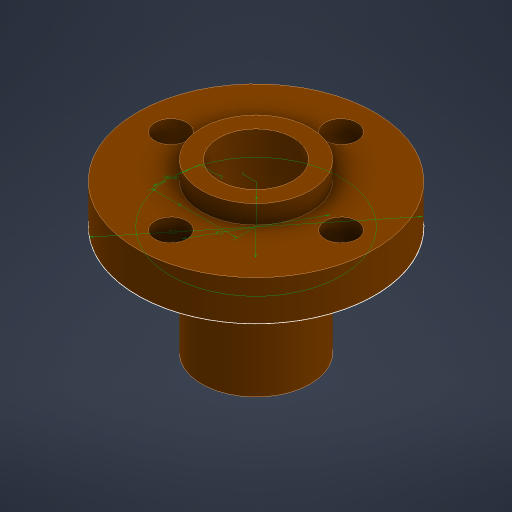
# Autodesk Inventor part: Leadscrew
Saved by Autodesk Inventor 2024.2 (Build 282272000, 272)
## iProperties
Created: 2024-10-02
Part Number: Leadscrew
Material: Generic
Document SubType Name: Modeling
Designer: jerem
Density: 1 g/cm^3
Appearance: Default
Author: jerem
Autodesk Inventor part; units mm, degrees
ref_plane "YZ Plane" through (0, 0, 0) normal (1, 0, 0) x (0, 1, 0)
ref_plane "XZ Plane" through (0, 0, 0) normal (0, 1, 0) x (-1, 0, 0)
ref_plane "XY Plane" through (0, 0, 0) normal (0, 0, 1) x (1, 0, 0)
sketch "Sketch1" plane through (0, 0, 0) normal (0, 1, 0) x (-1, 0, 0)
  circle A0 centre (0, 0) radius 11.15
  circle A1 centre (0, 0) radius 3.5
  circle A2 centre (8, 0) radius 1.5
  line L0 (8, 0) -> (0, 0) construction
  circle A3 centre (0, 8) radius 1.5
  circle A4 centre (-8, 0) radius 1.5
  circle A5 centre (0, -8) radius 1.5
  circle A6 centre (0, 0) radius 5.1
  dimension "d0" = 22.3
  dimension "d1" = 7
  dimension "d2" = 3
  dimension "d3" = 8
  dimension "d6" = 360
  dimension "d8" = 10.2
  constraints: 7 centre point, 3 coincident, 2 end point, 1 horizontal, 9 other
  measures "d0" diameter of A0
  measures "d1" diameter of A1
  measures "d2" diameter of A2
  measures "d3" distance of L0.start L0.end
  measures "d8" diameter of A6
extrude "Extrusion1" add sketch "Sketch1" along normal blind 3.75 contours A0 | A6
extrude "Extrusion2" add sketch "Sketch1" along normal blind 1.75 from surface at 3.75 contours A6
extrude "Extrusion3" add sketch "Sketch1" against normal blind 10.25 contours A6
body "Solid1"
